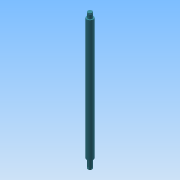
# Autodesk Inventor part: 中间传动轴
Saved by Autodesk Inventor 2015 (Build 190159000, 159)
## iProperties
Created: 2017-05-25
Part Number: 中间传动轴
Material: 常规
Document SubType Name: Modeling
Designer: Administrator
Density: 1 g/cm^3
Appearance: 灰蓝色
Author: Administrator
Autodesk Inventor part; units mm, degrees
ref_plane "YZ Plane" through (0, 0, 0) normal (1, 0, 0) x (0, 1, 0)
ref_plane "XY Plane" through (0, 0, 0) normal (0, 0, 1) x (1, 0, 0)
sketch "草图1" plane through (0, 0, 0) normal (0, 0, 1) x (1, 0, 0)
  circle A0 centre (0, 0) radius 15
  dimension "d0" = 30
  constraints: 1 centre point, 1 coincident
  measures "d0" diameter of A0
extrude "拉伸1" add sketch "草图1" along normal mid plane 561.864
sketch "草图2" plane through (0, 0, 280.932) normal (0, 0, 1) x (1, 0, 0)
  circle A0 centre (0, 0) radius 10
  dimension "d3" = 20
  constraints: 1 centre point, 1 coincident
  measures "d3" diameter of A0
extrude "拉伸2" add sketch "草图2" along normal blind 23.97
ref_plane "工作平面1" through (0, -10, 280.932) normal (0, 1, 0) x (-1, 0, 0)
sketch "草图3" plane through (0, -10, 280.932) normal (0, 1, 0) x (-1, 0, 0)
  line L0 (-3, 13.385) -> (3, 13.385)
  line L1 (3, 13.385) -> (3, 5.385)
  line L2 (3, 5.385) -> (-3, 5.385)
  line L3 (-3, 5.385) -> (-3, 13.385)
  arc A0 (3, 13.385) -> (-3, 13.385) centre (0, 13.385) ccw
  arc A1 (-3, 5.385) -> (3, 5.385) centre (0, 5.385) ccw
  line L4 (15, 0) -> (-15, 0) projected
  line L5 (0, 0) -> (0, 30.5075)
  point P0 (0, -280.932)
  dimension "d6" = 30.5075
  dimension "d7" = 6
  dimension "d8" = 8
  dimension "d9" = 5.385
  constraints: 10 end point, 4 point on circle, 4 tangent, 2 centre point, 2 midpoint, 2 parallel, 1 horizontal, 1 perpendicular, 1 point on line, 1 vertical
  measures "d6" distance of L5.start L5.end
  measures "d7" distance of L1.end L2.end
  measures "d8" distance of L2.end L0.start
  measures "d9" distance between parallel lines of L4 L2
extrude "拉伸3" cut sketch "草图3" along normal blind 2.5
sketch "草图4" plane through (0, 0, 0) normal (0, 1, 0) x (-1, 0, 0)
  line L0 (-9.175, 299.702) -> (-11.2925, 299.702)
  line L1 (-11.2925, 299.702) -> (-11.2925, 300.902)
  line L2 (-11.2925, 300.902) -> (-9.175, 300.902)
  line L3 (-9.175, 300.902) -> (-9.175, 299.702)
  line L4 (0, 0) -> (0, 472.2352)
  line L5 (10, 304.902) -> (-10, 304.902) projected
  line L6 (0, -94.447) -> (0, 566.6823) projected
  dimension "d12" = 472.2352
  dimension "d13" = 9.175
  dimension "d14" = 1.2
  dimension "d15" = 4
  dimension "d16" = 2.1175
  constraints: 10 end point, 2 parallel, 1 horizontal, 1 perpendicular, 1 vertical
  measures "d12" distance of L4.start L4.end
  measures "d13" distance between parallel lines of L4 L3
  measures "d14" distance of L0.end L1.end
  measures "d15" distance between parallel lines of L5 L2
  measures "d16" distance of L0.start L0.end
revolve "旋转1" cut sketch "草图4" angle 360 about axis through (0, 0, -10) along (0, 0, 1)
chamfer "倒角1" distance 0.5 angle 45 1 edges at (-10, 0, 304.902)
sketch "草图5" plane through (0, 0, -280.932) normal (0, 0, -1) x (-1, 0, 0)
  circle A0 centre (0, 0) radius 10
  dimension "d21" = 20
  constraints: 1 centre point, 1 coincident
  measures "d21" diameter of A0
extrude "拉伸4" add sketch "草图5" along normal blind 41.61
sketch "草图6" plane through (0, -10, 280.932) normal (0, 1, 0) x (-1, 0, 0)
  line L0 (3, -593.069) -> (-3, -593.069)
  line L1 (-3, -593.069) -> (-3, -567.069)
  line L2 (-3, -567.069) -> (3, -567.069)
  line L3 (3, -567.069) -> (3, -593.069)
  arc A0 (-3, -593.069) -> (3, -593.069) centre (0, -593.069) ccw
  arc A1 (3, -567.069) -> (-3, -567.069) centre (0, -567.069) ccw
  line L4 (-10, -603.474) -> (10, -603.474) projected
  line L5 (0, -603.474) -> (0, -655.1956)
  line L6 (-15, -561.864) -> (15, -561.864) projected
  point P0 (0, -280.932)
  dimension "d24" = 6
  dimension "d25" = 26
  dimension "d26" = 5.205
  constraints: 10 end point, 4 point on circle, 4 tangent, 2 centre point, 2 midpoint, 2 parallel, 1 horizontal, 1 perpendicular, 1 point on line, 1 vertical
  measures "d24" distance of L1.end L2.end
  measures "d25" distance of L2.end L0.start
  measures "d26" distance between parallel lines of L6 L2
extrude "拉伸5" cut sketch "草图6" along normal blind 2.5
sketch "草图7" plane through (0, 0, 0) normal (0, 1, 0) x (-1, 0, 0)
  line L0 (14.9872, -318.542) -> (9.175, -318.542)
  line L1 (9.175, -318.542) -> (9.175, -317.342)
  line L2 (9.175, -317.342) -> (14.9872, -317.342)
  line L3 (14.9872, -317.342) -> (14.9872, -318.542)
  line L4 (-10, -322.542) -> (10, -322.542) projected
  line L5 (0, -322.542) -> (0, -326.842)
  point P0 (0, 0)
  dimension "d29" = 4.3
  dimension "d30" = 1.2
  dimension "d31" = 5.8122
  dimension "d32" = 4
  dimension "d33" = 9.175
  constraints: 10 end point, 2 parallel, 1 horizontal, 1 midpoint, 1 perpendicular, 1 vertical
  measures "d29" distance of L5.start L5.end
  measures "d30" distance of L2.end L0.start
  measures "d31" distance of L1.end L2.end
  measures "d32" distance between parallel lines of L4 L0
  measures "d33" distance between parallel lines of L5 L1
revolve "旋转2" cut sketch "草图7" angle 360 about axis through (0, 0, -322.542) along (0, 0, -1)
chamfer "倒角2" distance 1 angle 45 1 edges at (10, 0, -322.542)
